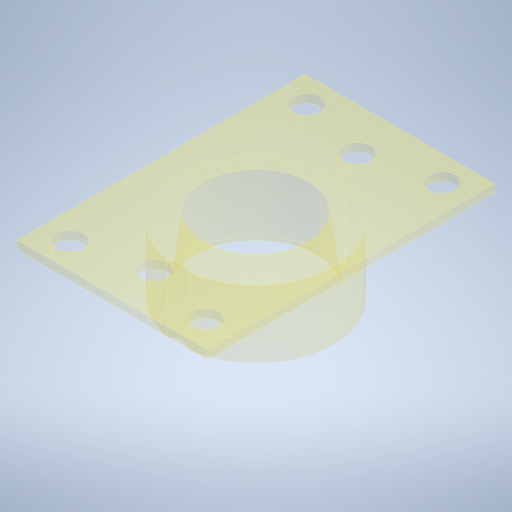
# Autodesk Inventor part: Gripper
Saved by Autodesk Inventor 2024 (Build 280153000, 153)
## iProperties
Created: 2023-12-19
Part Number: Gripper
Material: Thermoplastic Resin
Document SubType Name: Modeling
Designer: greg
Density: 1.28 g/cm^3
Appearance: Clear - Yellow
Author: greg
## iProperties of the stored document Gripper_3DPrint.ipt
Created: 2023-12-20
Part Number: Gripper_3DPrint
Material: Generic
Document SubType Name: Modeling
Designer: Greg
Density: 1 g/cm^3
Appearance: Default
Author: Greg
Autodesk Inventor part; units mm, degrees
ref_plane "YZ Plane" through (0, 0, 0) normal (1, 0, 0) x (0, 1, 0)
ref_plane "XZ Plane" through (0, 0, 0) normal (0, 1, 0) x (-1, 0, 0)
ref_plane "XY Plane" through (0, 0, 0) normal (0, 0, 1) x (1, 0, 0)
sketch "Sketch1" plane through (0, 0, 0) normal (0, 0, 1) x (1, 0, 0)
  line L0 (0, 0) -> (0, 14.2875)
  line L1 (0, 14.2875) -> (9.8425, 14.2875) construction
  line L2 (9.8425, 14.2875) -> (14.605, 14.2875)
  line L3 (14.605, 14.2875) -> (14.605, 0)
  line L4 (14.605, 0) -> (11.43, 1.5875)
  line L5 (11.43, 1.5875) -> (9.8425, 14.2875)
  dimension "d1" = 19.685
  dimension "d2" = 1.5875
  dimension "d3" = 3.175
  dimension "d5" = 14.2875
  dimension "d6" = 12.7
  constraints: 12 end point, 1 horizontal, 1 horizontal alignment, 1 perpendicular, 1 point on line, 1 vertical
  measures "d1" diameter of L1.end L0
  measures "d2" horizontal distance of L1.end L4.end
  measures "d3" horizontal distance of L3.end L4.end
  measures "d5" distance of L2.end L3.end
  measures "d6" vertical distance of L4.end L1.end
revolve "Revolution1" add sketch "Sketch1" angle 360 about axis through (0, 0, 0) along (0, 1, 0)
sketch "Sketch2" plane through (0, 14.2875, 0) normal (0, 1, 0) x (1, 0, 0)
  line L0 (17.78, -26.9875) -> (-17.78, -26.9875)
  line L1 (-17.78, -26.9875) -> (-17.78, 26.9875)
  line L2 (-17.78, 26.9875) -> (17.78, 26.9875)
  line L3 (17.78, 26.9875) -> (17.78, -26.9875)
  line L4 (17.78, -26.9875) -> (-17.78, 26.9875) construction
  line L5 (-17.78, -26.9875) -> (17.78, 26.9875) construction
  circle A0 centre (0, 0) radius 14.605 projected
  point P0 (0, -14.605)
  point P1 (-14.605, 0)
  dimension "d9" = 3.175
  dimension "d22" = 53.975
  constraints: 12 end point, 2 midpoint, 2 parallel, 2 point on circle, 1 horizontal, 1 horizontal alignment, 1 perpendicular, 1 vertical alignment
  measures "d9" distance from line of L1 A0.end
  measures "d22" distance of L0.end L1.end
extrude "Extrusion1" add sketch "Sketch2" against normal blind 1.5875
sketch "Sketch3" plane through (-17.78, 14.2875, -26.9875) normal (0, 1, 0) x (1, 0, 0)
  line L0 (17.78, -46.0375) -> (17.78, -7.9375) construction
  line L1 (5.08, -49.2125) -> (30.48, -49.2125)
  line L2 (30.48, -49.2125) -> (30.48, -4.7625)
  line L3 (30.48, -4.7625) -> (5.08, -4.7625)
  line L4 (5.08, -4.7625) -> (5.08, -49.2125)
  line L5 (5.08, -49.2125) -> (30.48, -4.7625) construction
  line L6 (30.48, -49.2125) -> (5.08, -4.7625) construction
  point P0 (17.78, -26.9875)
  point P1 (17.78, -26.9875)
  dimension "d12" = 38.1
  dimension "d20" = 44.45
  dimension "d21" = 25.4
  constraints: 14 end point, 7 coincident, 3 midpoint, 2 parallel, 1 horizontal, 1 perpendicular, 1 vertical
  measures "d12" distance of L0.start L0.end
  measures "d20" distance of L1.end L2.end
  measures "d21" distance of L2.end L3.end
hole "Hole1" at (12.7, 14.2875, 22.225) at (12.7, 14.2875, -22.225) at (-12.7, 14.2875, -22.225) at (-12.7, 14.2875, 22.225) at (0, 14.2875, -19.05) at (0, 14.2875, 19.05) direction (0, -1, 0) diameter 5.1054 end through all clearance for "Flat Head Machine Screw (82)" size "#10" standard "Ansi Unified Screw Threads"
sketch "Sketch4" plane through (0, 12.7, 0) normal (0, -1, 0) x (1, 0, 0)
  circle A0 centre (0, 19.05) radius 2.5527 projected
  circle A1 centre (0, 19.05) radius 5.08
  circle A2 centre (0, -19.05) radius 2.5527 projected
  circle A3 centre (0, -19.05) radius 5.08
  point P0 (0, 0)
  dimension "d23" = 10.16
  constraints: 2 centre point, 2 coincident, 1 equal radius
  measures "d23" diameter of A1
extrude "Extrusion2" cut sketch "Sketch4" along normal up to surface
body "Solid1"
